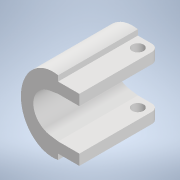
# Autodesk Inventor part: Falange proxima
Saved by Autodesk Inventor 2020 (Build 240168000, 168)
## iProperties
Created: 2021-08-19
Part Number: Falange proxima
Material: Generic
Document SubType Name: Modeling
Designer: chalo
Density: 1 g/cm^3
Appearance: Default
Author: chalo
Autodesk Inventor part; units mm, degrees
ref_plane "YZ Plane" through (0, 0, 0) normal (1, 0, 0) x (0, 1, 0)
ref_plane "XZ Plane" through (0, 0, 0) normal (0, 1, 0) x (-1, 0, 0)
ref_plane "XY Plane" through (0, 0, 0) normal (0, 0, 1) x (1, 0, 0)
sketch "Sketch1" plane through (0, 0, 0) normal (0, 0, 1) x (1, 0, 0)
  line L0 (3, 9.6082) -> (-3, 9.6082)
  line L1 (-3, 9.6082) -> (-3, 12.6082)
  line L2 (-3, 12.6082) -> (3, 12.6082)
  line L3 (3, 12.6082) -> (3, 9.6082)
  line L4 (-4.5, 3.8041) -> (5.5, 3.8041) construction
  line L5 (-3, -2) -> (3, -2) construction
  line L6 (-3, -2) -> (-3, -5)
  line L7 (-3, -5) -> (3, -5)
  line L8 (3, -5) -> (3, -2)
  line L9 (3, -2) -> (-3, -2)
  line L10 (-3, 12.6082) -> (-3, 14.1572)
  line L11 (-3, -5) -> (-3, -6.549)
  line L12 (-3, -2) -> (-5.3558, -1.6289)
  line L13 (-3, 9.6082) -> (-5.3558, 9.2371)
  ellipse E0 centre (-4.5, 3.8041) end of major axis (-4.5, -6.6959) minor radius 9 (3, -2) -> (3, 9.6082) ccw projected
  arc A0 (2.7798, 2) -> (2.7798, 5.6082) centre (-4.5, 3.8041) ccw projected
  line L14 (2.7798, 2) -> (3, 2) projected
  line L15 (3, 2) -> (3, -2) projected
  line L16 (3, 9.6082) -> (3, 5.6082) projected
  line L17 (3, 5.6082) -> (2.7798, 5.6082) projected
  ellipse E1 centre (-4.5, 3.8041) end of major axis (-4.5, -6.6959) minor radius 9 (3, -2) -> (3, 9.6082) ccw projected
  arc A1 (2.7798, 2) -> (2.7798, 5.6082) centre (-4.5, 3.8041) ccw projected
  line L18 (2.7798, 2) -> (3, 2) projected
  line L19 (3, 2) -> (3, -2) projected
  line L20 (3, 9.6082) -> (3, 5.6082) projected
  line L21 (3, 5.6082) -> (2.7798, 5.6082) projected
  arc A2 (-5.5, 9.2124) -> (-5.5, -1.6042) centre (-4.5, 3.8041) ccw projected
  line L22 (-5.5, 14.2391) -> (-5.5, 9.2124) projected
  ellipse E2 centre (-4.5, 3.8041) end of major axis (-4.5, -6.6959) minor radius 9 (-5.5, 14.2391) -> (-5.5, -6.6309) ccw projected
  line L23 (-5.5, -1.6042) -> (-5.5, -6.6309) projected
  line L24 (3, -2) -> (-3, -2) projected
  line L25 (-3, -2) -> (-3, -1.4874) projected
  arc A3 (-5.5, -1.6042) -> (-3, -1.4874) centre (-4.5, 3.8041) ccw projected
  arc A4 (-5.5, -1.6042) -> (-3, -1.4874) centre (-4.5, 3.8041) ccw projected
  ellipse E3 centre (-4.5, 3.8041) end of major axis (-4.5, -6.6959) minor radius 9 (-5.5, -6.6309) -> (3, -2) ccw projected
  line L26 (-5.5, -1.6042) -> (-5.5, -6.6309) projected
  line L27 (3, -2) -> (-3, -2) projected
  line L28 (-3, -2) -> (-3, -1.4874) projected
  ellipse E4 centre (-4.5, 3.8041) end of major axis (-4.5, -6.6959) minor radius 9 (-5.5, -6.6309) -> (3, -2) ccw projected
  line L29 (-5.5, -1.6042) -> (-5.5, -6.6309) projected
  ellipse E5 centre (-4.5, 3.8041) end of major axis (-4.5, -6.6959) minor radius 9 (3, 9.6082) -> (-5.5, 14.2391) ccw projected
  ellipse E6 centre (-4.5, 3.8041) end of major axis (-4.5, -6.6959) minor radius 9 (-5.5, 14.2391) -> (-5.5, -6.6309) ccw projected
  spline S0 degree 3 poles (-5.5, 9.2124) (-5.8842, 9.1414) (-6.264, 9.0282) (-7.2994, 8.5945) (-7.9078, 8.1744) (-8.8686, 7.2136) (-9.29, 6.6046) (-9.856, 5.2532) (-10, 4.5099) (-10, 3.0983) (-9.856, 2.355) (-9.29, 1.0036) (-8.8686, 0.3946) (-7.9078, -0.5662) (-7.2994, -0.9863) (-6.264, -1.42) (-5.8842, -1.5332) (-5.5, -1.6042) knots 0.098778 0.098778 0.098778 0.098778 0.212477 0.212477 0.424954 0.424954 0.636683 0.636683 0.848412 0.848412 1.06014 1.06014 1.271869 1.271869 1.484346 1.484346 1.598045 1.598045 1.598045 1.598045 projected
  arc A5 (-3, 9.0956) -> (-5.5, 9.2124) centre (-4.5, 3.8041) ccw projected
  point P0 (0, 0)
  point P1 (0.4043, -5)
  point P2 (0.4043, 12.6082)
  dimension "d0" = 6
  dimension "d1" = 3
  dimension "d2" = 10
  constraints: 28 end point, 3 symmetric about line, 2 horizontal, 2 parallel, 1 collinear, 1 perpendicular, 1 point on line, 1 vertical, 9 other
  measures "d0" distance of L1.end L2.end
  measures "d1" distance of L0.end L1.end
  measures "d2" distance of L4.start L4.end
extrude "Extrusion1" add sketch "Sketch1" along normal blind 18 and the other way blind 6.5 contours E5 L2 L3 | L0 L1 L2 E5 | L13 A5 L22 E5 L10 L1 | E3 L7 L6 L9 | L8 L7 E3 | L6 L11 E3 L23 A3 L12 | A2 L23 E2 L22
sketch "Sketch2" plane through (-3, 12.6082, 18) normal (0, 1, 0) x (1, 0, 0)
  circle A0 centre (3, 21.5) radius 1.6 projected
  point P0 (3, 18)
extrude "Extrusion2" cut sketch "Sketch2" against normal through all
fillet "Fillet1" radius 2 2 edges at (3, 11.1082, -6.5) (3, -3.5, -6.5)
sketch "Sketch6" plane through (0, 0, -6.5) normal (0, 0, -1) x (-1, 0, 0)
  ellipse E0 centre (4.5, 3.8041) end of major axis (4.5, -6.6959) minor radius 9 (3, -6.549) -> (3, 14.1572) ccw projected
  line L0 (3, 12.6082) -> (-1, 12.6082) projected
  line L1 (-1, 9.6082) -> (-1, 12.6082) projected
  line L2 (-1, 9.6082) -> (3, 9.6082) projected
  arc A0 (5.3558, -1.6289) -> (5.3558, 9.2371) centre (4.5, 3.8041) ccw projected
  line L3 (3, -2) -> (-1, -2) projected
  line L4 (4.5, 3.8041) -> (19.5, 3.8041)
  ellipse E1 centre (4.5, 3.8041) end of major axis (4.5, -6.6959) minor radius 9 (3, -6.549) -> (3, 14.1572) ccw projected
  line L5 (13.3352, 1.8041) -> (7.3352, 1.8041)
  line L6 (7.3352, 1.8041) -> (7.3352, -1.6959)
  line L7 (7.3352, -1.6959) -> (13.3352, -1.6959)
  line L8 (13.3352, -1.6959) -> (13.3352, 1.8041)
  line L9 (13.3352, 5.8041) -> (7.3352, 5.8041)
  line L10 (7.3352, 5.8041) -> (7.3352, 9.3041)
  line L11 (7.3352, 9.3041) -> (13.3352, 9.3041)
  line L12 (13.3352, 9.3041) -> (13.3352, 5.8041)
  line L13 (-1, -5) -> (-1, -2) projected
  line L14 (-1, -5) -> (3, -5) projected
  line L15 (3, 9.6082) -> (5.3558, 9.2371) projected
  line L16 (5.3558, -1.6289) -> (3, -2) projected
  line L17 (3, -5) -> (3, -6.549) projected
  line L18 (3, 14.1572) -> (3, 12.6082) projected
  point P0 (0, 0)
  point P1 (5.5, 14.2391)
  point P2 (-3, -2)
  point P3 (-0.4043, -5)
  point P4 (-0.4043, 12.6082)
  dimension "d11" = 15
  dimension "d12" = 6
  dimension "d13" = 3.5
  dimension "d14" = 4
  constraints: 18 end point, 4 symmetric about line, 2 horizontal, 2 parallel, 1 perpendicular, 3 other
  measures "d11" distance of L4.start L4.end
  measures "d12" distance of L7.end L6.end
  measures "d13" distance of L5.end L6.end
  measures "d14" distance between parallel lines of L9 L5
extrude "Extrusion3" add sketch "Sketch6" along normal blind 6 contours L7 L6 A0 L5 E0 | E0 L8 L7 | A0 L6 L5 | L9 A0 L10 L11 E0 | E0 L11 L12 | L9 L10 A0
fillet "Fillet2" radius 2 2 edges at (-8.7042, 7.3502, -6.5) (-8.7042, 0.258, -6.5)
sketch "Sketch7" plane through (-13.3352, 9.3041, -6.5) normal (0, 1, 0) x (1, 0, 0)
  line L0 (10.3352, 0) -> (1.1687, 0) projected
  line L1 (0, 0) -> (3.7118, 0) projected
  line L2 (0, 0) -> (0, 6) projected
  line L3 (0, 6) -> (6, 6) projected
  line L4 (6, 0) -> (6, 6) projected
  line L5 (6, 0) -> (6, 2) projected
  circle A0 centre (3, 3) radius 1.6
  point P0 (13.3352, -6.5)
  point P1 (0, 3)
  point P2 (3, 6)
  dimension "d19" = 3.2
  constraints: 2 midpoint, 1 centre point, 1 horizontal alignment, 1 vertical alignment
  measures "d19" diameter of A0
extrude "Extrusion4" cut sketch "Sketch7" against normal through all contours A0
fillet "Fillet4" radius 1 2 edges at (-12.8861, -0.0074, -6.5) (-12.8861, 7.6156, -6.5)
body "Solid1"
